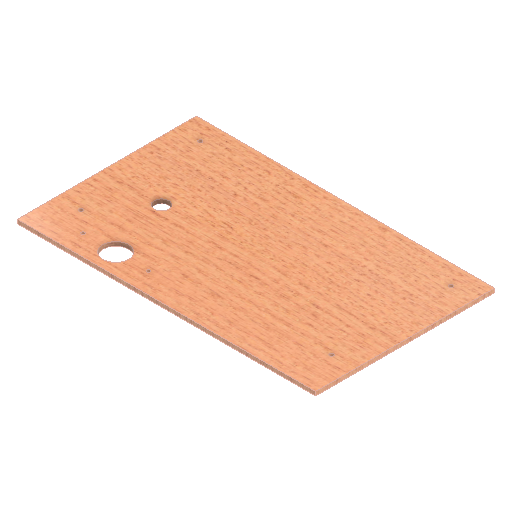
# Autodesk Inventor part: Upper
Saved by Autodesk Inventor 2025.2 (Build 292293000, 293)
## iProperties
Created: 2025-12-08
Part Number: Upper
Material: Generic
Document SubType Name: Modeling
Designer: hazem
Density: 1 g/cm^3
Appearance: Red Oak - Stained Light Medium Gloss
Author: hazem
Autodesk Inventor part; units mm, degrees
ref_plane "YZ Plane" through (0, 0, 0) normal (1, 0, 0) x (0, 1, 0)
ref_plane "XZ Plane" through (0, 0, 0) normal (0, 1, 0) x (-1, 0, 0)
ref_plane "XY Plane" through (0, 0, 0) normal (0, 0, 1) x (1, 0, 0)
sketch "Sketch1" plane through (0, 0, 0) normal (0, 1, 0) x (-1, 0, 0)
  line L0 (82.8007, 39.5361) -> (82.8007, -136.4639)
  line L1 (82.8007, -140.4639) -> (-217.1993, -140.4639)
  line L2 (-217.1993, -140.4639) -> (-217.1993, 35.5361)
  circle A0 centre (4.8007, 18.5361) radius 3.75
  circle A1 centre (-3.9493, 18.5361) radius 1.5
  circle A2 centre (13.5507, 18.5361) radius 1.5
  line L3 (4.8007, 22.2861) -> (4.8007, 14.7861) construction
  line L4 (-217.1993, 39.5361) -> (82.8007, 39.5361)
  line L5 (82.8007, -136.4639) -> (67.8007, -136.4639)
  line L6 (67.8007, -136.4639) -> (67.8007, -140.4639)
  line L7 (82.8007, -136.4639) -> (82.8007, -140.4639)
  line L8 (52.8007, -136.4639) -> (52.8007, -140.4639)
  line L9 (52.8007, -136.4639) -> (37.8007, -136.4639)
  line L10 (37.8007, -136.4639) -> (37.8007, -140.4639)
  line L11 (22.8007, -136.4639) -> (22.8007, -140.4639)
  line L12 (22.8007, -136.4639) -> (7.8007, -136.4639)
  line L13 (7.8007, -136.4639) -> (7.8007, -140.4639)
  line L14 (-7.1993, -136.4639) -> (-7.1993, -140.4639)
  line L15 (-7.1993, -136.4639) -> (-22.1993, -136.4639)
  line L16 (-22.1993, -136.4639) -> (-22.1993, -140.4639)
  line L17 (-37.1993, -136.4639) -> (-37.1993, -140.4639)
  line L18 (-37.1993, -136.4639) -> (-52.1993, -136.4639)
  line L19 (-52.1993, -136.4639) -> (-52.1993, -140.4639)
  line L20 (-67.1993, -136.4639) -> (-67.1993, -140.4639)
  line L21 (-67.1993, -136.4639) -> (-82.1993, -136.4639)
  line L22 (-82.1993, -136.4639) -> (-82.1993, -140.4639)
  line L23 (-97.1993, -136.4639) -> (-97.1993, -140.4639)
  line L24 (-97.1993, -136.4639) -> (-112.1993, -136.4639)
  line L25 (-112.1993, -136.4639) -> (-112.1993, -140.4639)
  line L26 (-127.1993, -136.4639) -> (-127.1993, -140.4639)
  line L27 (-127.1993, -136.4639) -> (-142.1993, -136.4639)
  line L28 (-142.1993, -136.4639) -> (-142.1993, -140.4639)
  line L29 (-157.1993, -136.4639) -> (-157.1993, -140.4639)
  line L30 (-157.1993, -136.4639) -> (-172.1993, -136.4639)
  line L31 (-172.1993, -136.4639) -> (-172.1993, -140.4639)
  line L32 (-187.1993, -136.4639) -> (-187.1993, -140.4639)
  line L33 (-187.1993, -136.4639) -> (-202.1993, -136.4639)
  line L34 (-202.1993, -136.4639) -> (-202.1993, -140.4639)
  line L35 (-217.1993, 35.5361) -> (-202.1993, 35.5361)
  line L36 (-202.1993, 35.5361) -> (-202.1993, 39.5361)
  line L37 (-217.1993, 35.5361) -> (-217.1993, 39.5361)
  line L38 (-172.1993, 35.5361) -> (-172.1993, 39.5361)
  line L39 (-187.1993, 35.5361) -> (-172.1993, 35.5361)
  line L40 (-187.1993, 35.5361) -> (-187.1993, 39.5361)
  line L41 (-142.1993, 35.5361) -> (-142.1993, 39.5361)
  line L42 (-157.1993, 35.5361) -> (-142.1993, 35.5361)
  line L43 (-157.1993, 35.5361) -> (-157.1993, 39.5361)
  line L44 (-112.1993, 35.5361) -> (-112.1993, 39.5361)
  line L45 (-127.1993, 35.5361) -> (-112.1993, 35.5361)
  line L46 (-127.1993, 35.5361) -> (-127.1993, 39.5361)
  line L47 (-82.1993, 35.5361) -> (-82.1993, 39.5361)
  line L48 (-97.1993, 35.5361) -> (-82.1993, 35.5361)
  line L49 (-97.1993, 35.5361) -> (-97.1993, 39.5361)
  line L50 (-52.1993, 35.5361) -> (-52.1993, 39.5361)
  line L51 (-67.1993, 35.5361) -> (-52.1993, 35.5361)
  line L52 (-67.1993, 35.5361) -> (-67.1993, 39.5361)
  line L53 (-22.1993, 35.5361) -> (-22.1993, 39.5361)
  line L54 (-37.1993, 35.5361) -> (-22.1993, 35.5361)
  line L55 (-37.1993, 35.5361) -> (-37.1993, 39.5361)
  line L56 (7.8007, 35.5361) -> (7.8007, 39.5361)
  line L57 (-7.1993, 35.5361) -> (7.8007, 35.5361)
  line L58 (-7.1993, 35.5361) -> (-7.1993, 39.5361)
  line L59 (37.8007, 35.5361) -> (37.8007, 39.5361)
  line L60 (22.8007, 35.5361) -> (37.8007, 35.5361)
  line L61 (22.8007, 35.5361) -> (22.8007, 39.5361)
  line L62 (67.8007, 35.5361) -> (67.8007, 39.5361)
  line L63 (52.8007, 35.5361) -> (67.8007, 35.5361)
  line L64 (52.8007, 35.5361) -> (52.8007, 39.5361)
  line L65 (-217.1993, -140.4639) -> (-213.1993, -140.4639)
  line L66 (-213.1993, -140.4639) -> (-213.1993, -125.4639)
  line L67 (-213.1993, -125.4639) -> (-217.1993, -125.4639)
  line L68 (-217.1993, -125.4639) -> (-217.1993, -140.4639)
  line L69 (-213.1993, -110.4639) -> (-213.1993, -95.4639)
  line L70 (-217.1993, -110.4639) -> (-213.1993, -110.4639)
  line L71 (-213.1993, -95.4639) -> (-217.1993, -95.4639)
  line L72 (-213.1993, -80.4639) -> (-213.1993, -65.4639)
  line L73 (-217.1993, -80.4639) -> (-213.1993, -80.4639)
  line L74 (-213.1993, -65.4639) -> (-217.1993, -65.4639)
  line L75 (-213.1993, -50.4639) -> (-213.1993, -35.4639)
  line L76 (-217.1993, -50.4639) -> (-213.1993, -50.4639)
  line L77 (-213.1993, -35.4639) -> (-217.1993, -35.4639)
  line L78 (-213.1993, -20.4639) -> (-213.1993, -5.4639)
  line L79 (-217.1993, -20.4639) -> (-213.1993, -20.4639)
  line L80 (-213.1993, -5.4639) -> (-217.1993, -5.4639)
  line L81 (-213.1993, 9.5361) -> (-213.1993, 24.5361)
  line L82 (-217.1993, 9.5361) -> (-213.1993, 9.5361)
  line L83 (-213.1993, 24.5361) -> (-217.1993, 24.5361)
  line L84 (82.8007, 39.5361) -> (78.8007, 39.5361)
  line L85 (78.8007, 39.5361) -> (78.8007, 24.5361)
  line L86 (78.8007, 24.5361) -> (82.8007, 24.5361)
  line L87 (82.8007, 24.5361) -> (82.8007, 39.5361)
  line L88 (78.8007, 9.5361) -> (78.8007, -5.4639)
  line L89 (78.8007, -5.4639) -> (82.8007, -5.4639)
  line L90 (82.8007, 9.5361) -> (78.8007, 9.5361)
  line L91 (78.8007, -20.4639) -> (78.8007, -35.4639)
  line L92 (78.8007, -35.4639) -> (82.8007, -35.4639)
  line L93 (82.8007, -20.4639) -> (78.8007, -20.4639)
  line L94 (78.8007, -50.4639) -> (78.8007, -65.4639)
  line L95 (78.8007, -65.4639) -> (82.8007, -65.4639)
  line L96 (82.8007, -50.4639) -> (78.8007, -50.4639)
  line L97 (78.8007, -80.4639) -> (78.8007, -95.4639)
  line L98 (78.8007, -95.4639) -> (82.8007, -95.4639)
  line L99 (82.8007, -80.4639) -> (78.8007, -80.4639)
  line L100 (78.8007, -110.4639) -> (78.8007, -125.4639)
  line L101 (78.8007, -125.4639) -> (82.8007, -125.4639)
  line L102 (82.8007, -110.4639) -> (78.8007, -110.4639)
  circle A3 centre (22.8007, -45.4639) radius 7.5
  circle A4 centre (58.8007, -0.4639) radius 2 projected
  circle A5 centre (58.8007, -120.4639) radius 2 projected
  circle A6 centre (58.8007, -0.4639) radius 2
  circle A7 centre (58.8007, -120.4639) radius 2
  circle A8 centre (-193.1993, -0.4639) radius 2 projected
  circle A9 centre (-193.1993, -120.4639) radius 2 projected
  point P0 (0, 0)
  point P1 (82.8007, -125.4639)
  point P2 (82.8007, -95.4639)
  point P3 (82.8007, -65.4639)
  point P4 (82.8007, -35.4639)
  point P5 (82.8007, -5.4639)
  point P6 (82.8007, 24.5361)
  point P7 (78.8007, 39.5361)
  point P8 (67.8007, 39.5361)
  point P9 (52.8007, 39.5361)
  point P10 (37.8007, 39.5361)
  point P11 (22.8007, 39.5361)
  point P12 (7.8007, 39.5361)
  point P13 (-7.1993, 39.5361)
  point P14 (-22.1993, 39.5361)
  point P15 (-37.1993, 39.5361)
  point P16 (-52.1993, 39.5361)
  point P17 (-67.1993, 39.5361)
  point P18 (-112.1993, 39.5361)
  point P19 (-172.1993, 39.5361)
  point P20 (-202.1993, -140.4639)
  point P21 (-187.1993, -140.4639)
  point P22 (-172.1993, -140.4639)
  point P23 (-157.1993, -140.4639)
  point P24 (-142.1993, -140.4639)
  dimension "d1" = 7.5
  dimension "d2" = 3
  dimension "d3" = 8.75
  dimension "d24" = 4
  dimension "d25" = 15
  dimension "d28" = 30
  dimension "d33" = 4
  dimension "d34" = 15
  dimension "d37" = 30
  dimension "d42" = 4
  dimension "d43" = 15
  dimension "d46" = 30
  dimension "d51" = 4
  dimension "d52" = 15
  dimension "d55" = 30
  dimension "d60" = 15
  dimension "d61" = 85
  dimension "d62" = 60
  constraints: 202 end point, 74 horizontal alignment, 44 parallel, 18 collinear, 7 vertical, 6 centre point, 4 horizontal, 3 coincident, 3 equal radius, 2 perpendicular, 2 point on circle, 1 midpoint, 79 other
  measures "d1" diameter of A0
  measures "d2" diameter of A2
  measures "d3" distance of A0.centre A2.centre
  measures "d25" distance of L0.end L5.end
  measures "d28" distance of L0.end L8.start
  measures "d34" distance of L2.end L35.end
  measures "d37" distance of L35.end L38.start
  measures "d42" distance of L67.end L66.end
  measures "d43" distance of L66.end L65.end
  measures "d46" distance of L65.end L69.start
  measures "d51" distance of L86.end L85.end
  measures "d52" distance of L85.end L84.end
  measures "d55" distance of L84.end L88.start
  measures "d60" diameter of A3
  measures "d62" distance from line of L0 A3.centre
extrude "Extrusion1" add sketch "Sketch1" along normal blind 4
sketch "Sketch2" plane through (0, 4, 0) normal (0, 1, 0) x (1, 0, 0)
  circle A0 centre (-4.8007, -18.5361) radius 13
  circle A1 centre (-4.8007, -18.5361) radius 3.75 projected
  circle A2 centre (-37.8007, -18.5361) radius 1.75
  circle A3 centre (28.1993, -18.5361) radius 1.75
  point P0 (0, 0)
  dimension "d63" = 26
  dimension "d64" = 3.5
  dimension "d65" = 3.5
  dimension "d66" = 33
  dimension "d67" = 33
  constraints: 3 centre point, 2 horizontal alignment, 1 concentric
  measures "d63" diameter of A0
  measures "d64" diameter of A2
  measures "d65" diameter of A3
  measures "d66" distance of A2.centre A0.centre
  measures "d67" distance of A3.centre A0.centre
extrude "Extrusion2" cut sketch "Sketch2" against normal through all contours A0 | A1 | A2 | A3
equation "\"d24\" = WoodThickness"
equation "\"d28\" = 2 * d25"
equation "\"d33\" = WoodThickness"
equation "\"d34\" = d25"
equation "\"d37\" = 2 * d34"
equation "\"d42\" = WoodThickness"
equation "\"d46\" = 2 * d43"
equation "\"d51\" = WoodThickness"
equation "\"d55\" = 2 * d52"
equation "\"WoodThickness\" = 4"
body "Solid1"
